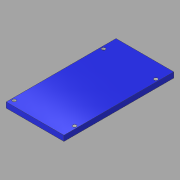
# Autodesk Inventor part: Arduino Mount
Saved by Autodesk Inventor 2017 (Build 210142000, 142)
## iProperties
Created: 2016-12-06
Part Number: Arduino Mount
Material: Polystyrene, High Impact
Document SubType Name: Modeling
Designer: qupec
Density: 1.022 g/cm^3
Appearance: Smooth - White
Author: qupec
Autodesk Inventor part; units mm, degrees
ref_plane "YZ Plane" through (0, 0, 0) normal (1, 0, 0) x (0, 1, 0)
ref_plane "XZ Plane" through (0, 0, 0) normal (0, 1, 0) x (-1, 0, 0)
ref_plane "XY Plane" through (0, 0, 0) normal (0, 0, 1) x (1, 0, 0)
sketch "Sketch1" plane through (0, 0, 0) normal (0, 1, 0) x (-1, 0, 0)
  line L0 (26.7081, 50.8) -> (-26.7081, 50.8)
  line L1 (-26.7081, 50.8) -> (-26.7081, -50.8)
  line L2 (-26.7081, -50.8) -> (26.7081, -50.8)
  line L3 (26.7081, -50.8) -> (26.7081, 50.8)
  point P0 (0, 0)
  dimension "d0" = 101.6
  dimension "d1" = 53.4162
  dimension "d2" = 26.7081
  dimension "d3" = 50.8
  constraints: 8 end point, 2 parallel, 1 horizontal, 1 perpendicular
  measures "d0" distance of L2.end L0.start
  measures "d1" distance of L0.start L0.end
  measures "d2" distance from line of point (0, 0) L1
  measures "d3" distance from line of point (0, 0) L0
extrude "Extrusion1" add sketch "Sketch1" along normal blind 5
sketch "Sketch3" plane through (0, 5, 0) normal (0, 1, 0) x (1, 0, 0)
  circle A0 centre (-24.1681, -45.9486) radius 1.5875
  line L0 (-26.7081, 50.8) -> (-26.7081, -50.8) projected
  circle A1 centre (24.1681, -38.4556) radius 1.5621
  line L1 (26.7081, -50.8) -> (26.7081, 50.8) projected
  circle A2 centre (-24.1681, 36.6776) radius 1.5621
  line L2 (26.7081, 50.8) -> (-26.7081, 50.8) projected
  circle A3 centre (24.1681, 36.6776) radius 1.5621
  line L3 (-26.7081, -50.8) -> (26.7081, -50.8) projected
  point P0 (0, 0)
  dimension "d6" = 3.175
  dimension "d7" = 2.54
  dimension "d9" = 3.1242
  dimension "d10" = 2.54
  dimension "d12" = 3.1242
  dimension "d13" = 2.54
  dimension "d14" = 14.1224
  dimension "d15" = 3.1242
  dimension "d16" = 14.1224
  dimension "d17" = 2.54
  dimension "d32" = 4.8514
  dimension "d36" = 75.1332
  constraints: 4 centre point
  measures "d6" diameter of A0
  measures "d7" distance from line of L0 A0.centre
  measures "d9" diameter of A1
  measures "d10" distance from line of L1 A1.centre
  measures "d12" diameter of A2
  measures "d13" distance from line of L0 A2.centre
  measures "d14" distance from line of L2 A2.centre
  measures "d15" diameter of A3
  measures "d16" distance from line of L2 A3.centre
  measures "d17" distance from line of L1 A3.centre
  measures "d32" distance from line of L3 A0.centre
  measures "d36" distance of A1.centre A3.centre
extrude "Extrusion4" cut sketch "Sketch3" against normal through all contours A0 | A1 | A2 | A3
equation "\"d2\" = 0.5 * d1"
equation "\"d3\" = 0.5 * d0"
equation "\"d9\" = d15"
body "Solid1"
